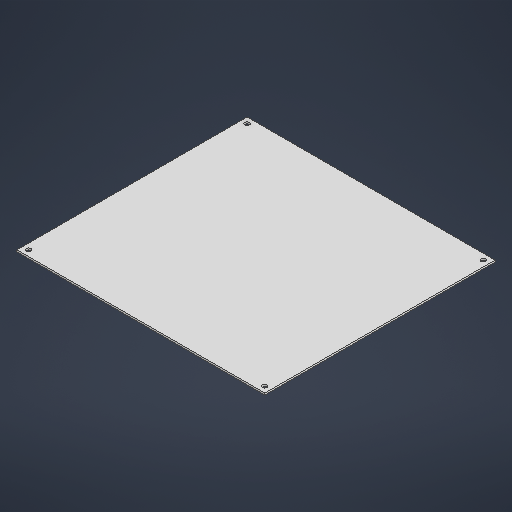
# Autodesk Inventor part: TapaLateral
Saved by Autodesk Inventor 2026.2 (Build 302298010, 298A)
## iProperties
Created: 2026-04-14
Part Number: TapaLateral
Material: Generic
Document SubType Name: Modeling
Designer: grego
Density: 1 g/cm^3
Appearance: Default
Author: grego
Autodesk Inventor part; units mm, degrees
ref_plane "YZ Plane" through (0, 0, 0) normal (1, 0, 0) x (0, 1, 0)
ref_plane "XZ Plane" through (0, 0, 0) normal (0, 1, 0) x (-1, 0, 0)
ref_plane "XY Plane" through (0, 0, 0) normal (0, 0, 1) x (1, 0, 0)
sketch "Sketch1" plane through (0, 0, 0) normal (0, 1, 0) x (-1, 0, 0)
  line L0 (210, 195) -> (-210, 195)
  line L1 (-210, 195) -> (-210, -195)
  line L2 (-210, -195) -> (210, -195)
  line L3 (210, -195) -> (210, 195)
  line L4 (210, 195) -> (-210, -195) construction
  line L5 (-210, 195) -> (210, -195) construction
  circle A0 centre (200, -185) radius 4
  circle A1 centre (-200, -185) radius 4
  circle A2 centre (-200, 185) radius 4
  circle A3 centre (200, 185) radius 4
  point P0 (0, 0)
  dimension "d0" = 420
  dimension "d1" = 390
  dimension "d3" = 8
  dimension "d4" = 8
  dimension "d5" = 8
  dimension "d6" = 8
  constraints: 12 end point, 4 centre point, 2 midpoint, 2 parallel, 1 horizontal, 1 perpendicular
  measures "d0" distance of L2.end L1.end
  measures "d1" distance of L1.end L0.end
  measures "d3" diameter of A0
  measures "d4" diameter of A1
  measures "d5" diameter of A2
  measures "d6" diameter of A3
extrude "Extrusion1" add sketch "Sketch1" along normal blind 3
body "Solid1"
